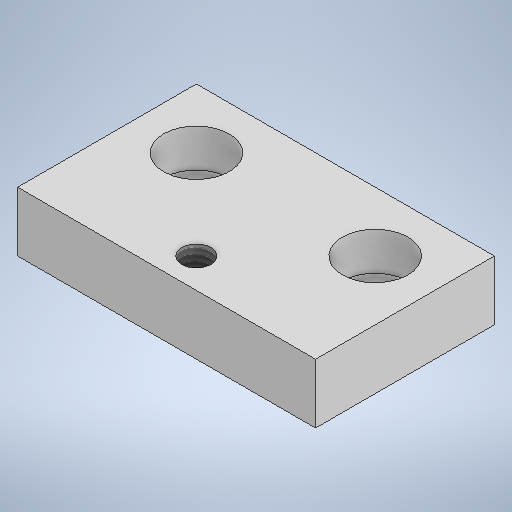
# Autodesk Inventor part: JH_Positionierungseinheit_Vertikalbegrenzung_int
Saved by Autodesk Inventor 2025.1 (Build 291241000, 241)
## iProperties
Created: 2025-05-23
Part Number: JH_Positionierungseinheit_Vertikalbegrenzung_int
Material: Generisch
Document SubType Name: Modeling
Designer: Jakob
Density: 1 g/cm^3
Appearance: Vorgabe
Author: Jakob
Autodesk Inventor part; units mm, degrees
ref_plane "YZ Plane" through (0, 0, 0) normal (1, 0, 0) x (0, 1, 0)
ref_plane "XZ Plane" through (0, 0, 0) normal (0, 1, 0) x (-1, 0, 0)
ref_plane "XY Plane" through (0, 0, 0) normal (0, 0, 1) x (1, 0, 0)
sketch "Skizze1" plane through (0, 0, 0) normal (0, 0, 1) x (1, 0, 0)
  line L0 (-25, 15) -> (25, 15)
  line L1 (25, 15) -> (25, -15)
  line L2 (25, -15) -> (-25, -15)
  line L3 (-25, -15) -> (-25, 15)
  line L4 (-25, 15) -> (25, -15) construction
  line L5 (25, 15) -> (-25, -15) construction
  point P0 (0, 0)
  dimension "d0" = 50
  dimension "d1" = 30
  constraints: 12 end point, 2 midpoint, 2 parallel, 1 horizontal, 1 perpendicular
  measures "d0" distance of L0.start L0.end
  measures "d1" distance of L0.end L1.end
extrude "Extrusion1" add sketch "Skizze1" along normal mid plane 10
sketch "Skizze3" plane through (0, 0, 5) normal (0, 0, 1) x (1, 0, 0)
  line L0 (-35, 0) -> (35, 0) projected
  line L1 (25, 15) -> (-25, 15) projected
  line L2 (0, -21) -> (0, 21) projected
  line L3 (0, 21) -> (0, -21) projected
  point P0 (0, 0)
  point P1 (0, -10)
  point P2 (15, 5)
  dimension "d6" = 25
  dimension "d16" = 10
  dimension "d31" = 15
  constraints: 1 point on line
  measures "d6" distance from line of L1 point (0, -10)
  measures "d16" distance from line of L1 point (15, 5)
  measures "d31" distance from line of L3 point (15, 5)
hole "Bohrung1" at (0, -10, 5) direction (0, 0, -1) diameter 4.917 end through all thread size "M6x1" class "6H" standard "ISO Metric profile"
hole "Bohrung2" at (15, 5, 5) direction (0, 0, -1) diameter 6.6 end through all counterbore diameter 11 counterbore depth 6.4 clearance for "Sechskantkopfschraube DIN EN 24017" size "M6" standard "DIN"
mirror "Spiegeln1" about plane through (0, 0, 0) normal (1, 0, 0) of "Bohrung2"
equation "\"d0\" = Länge_Vertikalbegrenzung"
equation "\"d1\" = Breite_Vertikalbegrenzung"
equation "\"d2\" = Tiefe_Vertikalbegrenzung"
equation "\"d6\" = Abstand_Bohrung_Madenschraube"
equation "\"d16\" = Abstand_Bohrungen_y"
equation "\"d31\" = Abstand_Bohrungen_x"
equation "\"Länge_Vertikalbegrenzung\" = 50"
equation "\"Breite_Vertikalbegrenzung\" = 30"
equation "\"Tiefe_Vertikalbegrenzung\" = 10"
equation "\"Abstand_Bohrung_Madenschraube\" = 25"
equation "\"Abstand_Bohrungen_x\" = 15"
equation "\"Abstand_Bohrungen_y\" = 10"
